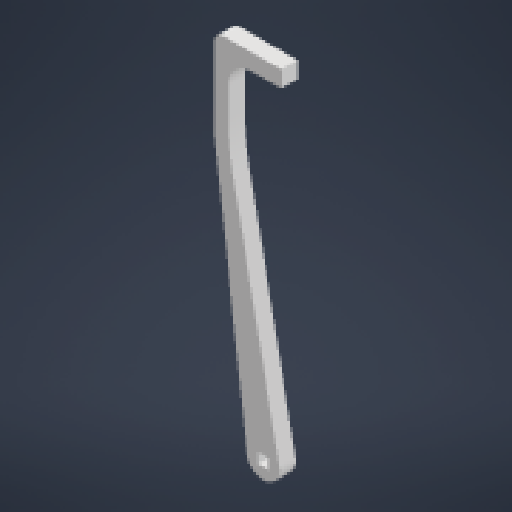
# Autodesk Inventor part: Arm
Saved by Autodesk Inventor 2025 (Build 290162000, 162)
## iProperties
Created: 2024-12-26
Part Number: Arm
Material: Типовые
Document SubType Name: Modeling
Designer: khrip
Density: 1 g/cm^3
Appearance: По умолчанию
Author: khrip
Autodesk Inventor part; units mm, degrees
ref_plane "YZ Plane" through (0, 0, 0) normal (1, 0, 0) x (0, 1, 0)
ref_plane "XZ Plane" through (0, 0, 0) normal (0, 1, 0) x (-1, 0, 0)
ref_plane "XY Plane" through (0, 0, 0) normal (0, 0, 1) x (1, 0, 0)
sketch "Эскиз1" plane through (0, 0, 0) normal (0, 0, 1) x (1, 0, 0)
  circle A0 centre (0.0899, -0.0505) radius 4 projected
  line L0 (-20.8576, 111.2941) -> (-20.8576, 149.3795)
  line L1 (-20.8576, 149.3795) -> (-6.2988, 149.3795)
  line L2 (7.9099, 149.3795) -> (-6.2988, 149.3795)
  line L3 (-14.8576, 142.2545) -> (7.9099, 142.2545)
  line L4 (-14.8576, 142.2545) -> (7.9099, 142.2545)
  line L5 (-14.8576, 109.9334) -> (-14.8576, 142.2545)
  circle A1 centre (0.0899, -0.0505) radius 7
  line L6 (-2.25, -2.25) -> (2.25, -2.25)
  line L7 (2.25, -2.25) -> (2.25, 2.25)
  line L8 (2.25, 2.25) -> (-2.25, 2.25)
  line L9 (-2.25, 2.25) -> (-2.25, -2.25)
  line L10 (-2.25, -2.25) -> (2.25, 2.25) construction
  line L11 (2.25, -2.25) -> (-2.25, 2.25) construction
  line L12 (7.9099, 142.2545) -> (7.9099, 149.3795)
  line L13 (-20.8576, 111.2941) -> (-6.8563, -0.9172)
  line L14 (-14.8576, 109.9334) -> (6.9529, 1.3278)
  point P0 (0, 0)
  dimension "d0" = 14
  dimension "d1" = 4.5
  dimension "d2" = 4.5
  constraints: 30 end point, 5 horizontal, 3 vertical, 2 midpoint, 2 parallel, 2 point on circle, 2 tangent, 1 centre point, 1 coincident, 1 perpendicular, 7 other
  measures "d0" diameter of A1
  measures "d1" distance of L8.end L7.end
  measures "d2" distance of L7.end L6.end
extrude "Выдавливание1" add sketch "Эскиз1" along normal blind 7 contours A0 | L0 L1 L2 L12 L3 L5 L14 A1 L13 | A1
fillet "Сопряжение1" radius 10 1 edges at (-14.8576, 142.2545, 3.5)
fillet "Сопряжение2" radius 4 1 edges at (-20.8576, 149.3795, 3.5)
fillet "Сопряжение3" radius 100 1 edges at (-14.8576, 109.9334, 3.5)
